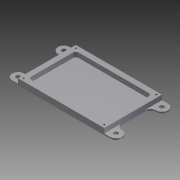
# Autodesk Inventor part: Base.Box.Base
Saved by Autodesk Inventor 2011 (Build 150239000, 239)
## iProperties
Created: 2011-05-11
Part Number: Base.Box.Base
Document SubType Name: Modeling
Designer: Rob
Density: 1 g/cm^3
Author: Rob
Autodesk Inventor part; units mm, degrees
ref_plane "YZ Plane" through (0, 0, 0) normal (1, 0, 0) x (0, 1, 0)
ref_plane "XZ Plane" through (0, 0, 0) normal (0, 1, 0) x (-1, 0, 0)
ref_plane "XY Plane" through (0, 0, 0) normal (0, 0, 1) x (1, 0, 0)
sketch "Sketch1" plane through (0, 0, 0) normal (0, 0, 1) x (1, 0, 0)
  line L0 (-83, 53) -> (83, 53) construction
  line L1 (83, 53) -> (83, -53) construction
  line L2 (83, -53) -> (-83, -53) construction
  line L3 (-83, -53) -> (-83, 53) construction
  line L4 (-83, -53) -> (83, 53) construction
  line L5 (83, -53) -> (-83, 53) construction
  line L6 (-91, 61) -> (91, 61)
  line L7 (91, 61) -> (91, -61)
  line L8 (91, -61) -> (-91, -61)
  line L9 (-91, -61) -> (-91, 61)
  line L10 (-91, 61) -> (91, -61) construction
  line L11 (-91, -61) -> (91, 61) construction
  line L12 (-91, 61) -> (-116, 61)
  line L13 (-116, 61) -> (-116, 36)
  line L14 (-116, 36) -> (-91, 36)
  line L15 (-91, 36) -> (-91, 61)
  line L16 (0, 0) -> (-160.1953, 0) construction
  line L17 (-91, -61) -> (-116, -61)
  line L18 (-116, -61) -> (-116, -36)
  line L19 (-116, -36) -> (-91, -36)
  line L20 (-91, -36) -> (-91, -61)
  line L21 (0, 0) -> (0, 107.5555) construction
  line L22 (91, -61) -> (91, 61)
  line L23 (91, 61) -> (116, 61)
  line L24 (116, 61) -> (116, 36)
  line L25 (116, 36) -> (91, 36)
  line L26 (91, 36) -> (91, 61)
  line L27 (91, -36) -> (91, -61)
  line L28 (91, -61) -> (116, -61)
  line L29 (116, -61) -> (116, -36)
  line L30 (116, -36) -> (91, -36)
  point P0 (0, 0)
  point P1 (0, 0)
  dimension "d0" = 166
  dimension "d1" = 106
  dimension "d2" = 8
  dimension "d3" = 8
  dimension "d4" = 25
  dimension "d5" = 25
  constraints: 62 end point, 9 symmetric about line, 6 parallel, 5 midpoint, 5 perpendicular, 3 horizontal, 1 coincident
  measures "d0" distance of L1.end L2.end
  measures "d1" distance of L0.end L1.end
  measures "d2" distance between parallel lines of L3 L9
  measures "d3" distance between parallel lines of L0 L6
  measures "d4" distance of L14.end L13.end
  measures "d5" distance of L12.end L13.end
extrude "Extrusion1" add sketch "Sketch1" along normal blind 3
sketch "Sketch2" plane through (0, 0, 3) normal (0, 0, 1) x (1, 0, 0)
  line L0 (-116, 61) -> (116, 61) projected
  line L1 (-116, 36) -> (-116, 61) projected
  line L2 (116, 61) -> (116, 36) projected
  circle A0 centre (-103.5, 48.5) radius 1
  line L3 (0, 0) -> (-24.3275, 0) construction
  line L4 (0, 0) -> (0, 26.5856) construction
  circle A1 centre (-103.5, -48.5) radius 1
  circle A2 centre (103.5, 48.5) radius 1
  circle A3 centre (103.5, -48.5) radius 1
  dimension "d8" = 2
  dimension "d9" = 12.5
  dimension "d10" = 12.5
  constraints: 4 centre point, 4 end point, 3 symmetric about line, 2 perpendicular, 3 other
  measures "d8" diameter of A0
  measures "d9" distance from line of L1 A0.centre
  measures "d10" distance from line of L0 A0.centre
hole "Hole1" at (-103.5, 48.5, 3) at (-103.5, -48.5, 3) at (103.5, -48.5, 3) at (103.5, 48.5, 3) direction (0, 0, -1) diameter 9 depth 8 tip angle 118 clearance for "Flat Head Machine Screw" size "M8" standard "Ansi Metric M Profile"
fillet "Fillet1" radius 12.5 12 edges at (116, 61, 1.5) (116, 36, 1.5) (91, 36, 1.5) (91, -36, 1.5) (116, -36, 1.5) (116, -61, 1.5) (-116, -61, 1.5) (-116, -36, 1.5) (-91, -36, 1.5) (-91, 36, 1.5) (-116, 36, 1.5) (-116, 61, 1.5)
sketch "Sketch3" plane through (0, 0, 3) normal (0, 0, 1) x (1, 0, 0)
  line L0 (103.5, -61) -> (-103.5, -61) projected
  line L1 (-103.5, 61) -> (103.5, 61) projected
  line L2 (-91, 61) -> (91, 61)
  line L3 (91, 61) -> (91, -61)
  line L4 (91, -61) -> (-91, -61)
  line L5 (-91, -61) -> (-91, 61)
  line L6 (-80, 50) -> (80, 50)
  line L7 (80, 50) -> (80, -50)
  line L8 (80, -50) -> (-80, -50)
  line L9 (-80, -50) -> (-80, 50)
  line L10 (-80, 50) -> (80, -50) construction
  line L11 (-80, -50) -> (80, 50) construction
  line L12 (-91, -23.5) -> (-91, 23.5) projected
  point P0 (0, 0)
  dimension "d19" = 100
  dimension "d20" = 160
  constraints: 20 end point, 4 parallel, 2 horizontal, 2 midpoint, 2 perpendicular, 2 point on line, 1 collinear
  measures "d19" distance of L8.end L6.start
  measures "d20" distance of L6.start L6.end
extrude "Extrusion2" add sketch "Sketch3" along normal blind 10
fillet "Fillet2" radius 6 4 edges at (-80, 50, 8) (-80, -50, 8) (80, -50, 8) (80, 50, 8)
sketch "Sketch6" plane through (0, 0, 13) normal (0, 0, 1) x (1, 0, 0)
  line L0 (-91, 61) -> (91, 61) projected
  line L1 (-91, -61) -> (-91, 61) projected
  circle A0 centre (-85, 55) radius 2
  line L2 (0, 0) -> (-11.4122, 0) construction
  line L3 (0, 0) -> (0, 13.6861) construction
  circle A1 centre (-85, -55) radius 2
  circle A2 centre (85, 55) radius 2
  circle A3 centre (85, -55) radius 2
  dimension "d33" = 4
  dimension "d34" = 6
  dimension "d35" = 6
  constraints: 4 centre point, 4 end point, 3 symmetric about line, 2 perpendicular, 3 other
  measures "d33" diameter of A0
  measures "d34" distance from line of L0 A0.centre
  measures "d35" distance from line of L1 A0.centre
hole "Hole2" at (-85, 55, 13) at (-85, -55, 13) at (85, -55, 13) at (85, 55, 13) direction (0, 0, -1) diameter 3.242 depth 8 tip angle 118 thread size "M4x0.7" class "6H" standard "ANSI Metric M Profile"
equation "\"d34\" = 1.5 * d33"
equation "\"d35\" = 1.5 * d33"
body "Solid1"
